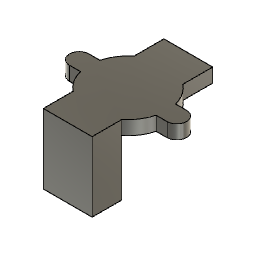
[new] Stepper Motor Cover v7 (Autodesk Fusion 360 design; units mm, degrees)
Autodesk Fusion 360 part; units mm, degrees
sketch "Sketch1" plane through (0, 0, 24.0553) normal (0, 0, 1) x (-1, 0, 0)
  line L0 (10.7499, 16.3506) -> (10.7499, 5.6583)
  line L1 (10.7499, 5.6583) -> (-6.7501, 5.6583)
  line L2 (-6.7501, 5.6583) -> (-6.7501, 16.3506)
  arc A0 (-11.5555, 23.7794) -> (-6.7501, 16.3506) centre (1.9999, 27.2794) ccw
  line L3 (-11.5555, 23.7794) -> (-15.5001, 23.7794)
  arc A1 (-15.5001, 30.7794) -> (-15.5001, 23.7794) centre (-15.5001, 27.2794) ccw
  line L4 (-15.5001, 30.7794) -> (-11.5555, 30.7794)
  arc A2 (-6.7501, 38.2081) -> (-11.5555, 30.7794) centre (1.9999, 27.2794) ccw
  line L5 (-6.7501, 38.2081) -> (-6.7501, 48.9005)
  line L6 (-6.7501, 48.9005) -> (10.7499, 48.9005)
  line L7 (10.7499, 48.9005) -> (10.7499, 38.2081)
  arc A3 (15.5554, 30.7794) -> (10.7499, 38.2081) centre (1.9999, 27.2794) ccw
  line L8 (15.5554, 30.7794) -> (19.4999, 30.7794)
  arc A4 (19.4999, 23.7794) -> (19.4999, 30.7794) centre (19.4999, 27.2794) ccw
  line L9 (19.4999, 23.7794) -> (15.5554, 23.7794)
  arc A5 (10.7499, 16.3506) -> (15.5554, 23.7794) centre (1.9999, 27.2794) ccw
  arc A6 (51.4999, 44.5294) -> (41.4999, 54.5294) centre (41.4999, 44.5294) ccw
  line L10 (41.4999, 54.5294) -> (-37.5001, 54.5294)
  arc A7 (-37.5001, 54.5294) -> (-47.5001, 44.5294) centre (-37.5001, 44.5294) ccw
  line L11 (-47.5001, 44.5294) -> (-47.5001, -34.4706)
  arc A8 (-47.5001, -34.4706) -> (-37.5001, -44.4706) centre (-37.5001, -34.4706) ccw
  line L12 (-37.5001, -44.4706) -> (41.4999, -44.4706)
  arc A9 (41.4999, -44.4706) -> (51.4999, -34.4706) centre (41.4999, -34.4706) ccw
  line L13 (51.4999, -34.4706) -> (51.4999, 44.5294)
  line L14 (42.9999, -37.9706) -> (-39.0001, -37.9706)
  line L15 (-39.0001, -37.9706) -> (-39.0001, 0.0294)
  line L16 (-39.0001, 0.0294) -> (42.9999, 0.0294)
  line L17 (42.9999, 0.0294) -> (42.9999, -37.9706)
  line L18 (10.7499, 48.9005) -> (10.7499, 38.2081)
  line L19 (-6.7501, 48.9005) -> (10.7499, 48.9005)
  line L20 (-6.7501, 38.2081) -> (-6.7501, 48.9005)
  arc A10 (-6.7501, 38.2081) -> (-11.5555, 30.7794) centre (1.9999, 27.2794) ccw
  arc A11 (15.5554, 30.7794) -> (10.7499, 38.2081) centre (1.9999, 27.2794) ccw
  line L21 (15.5554, 30.7794) -> (19.4999, 30.7794)
  arc A12 (19.4999, 23.7794) -> (19.4999, 30.7794) centre (19.4999, 27.2794) ccw
  line L22 (19.4999, 23.7794) -> (15.5554, 23.7794)
  arc A13 (15.5524, 23.7794) -> (15.5583, 30.7794) centre (1.9999, 27.2908) ccw
  line L23 (15.5524, 23.7794) -> (19.4999, 23.7794)
  arc A14 (19.4999, 23.7794) -> (19.4999, 30.7794) centre (19.4999, 27.2794) ccw
  line L24 (19.4999, 30.7794) -> (15.5583, 30.7794)
  circle A15 centre (19.4999, 27.2794) radius 2
  arc A16 (-11.5585, 30.7794) -> (-11.5526, 23.7794) centre (1.9999, 27.2908) ccw
  line L25 (-11.5585, 30.7794) -> (-15.5001, 30.7794)
  arc A17 (-15.5001, 30.7794) -> (-15.5001, 23.7794) centre (-15.5001, 27.2794) ccw
  line L26 (-15.5001, 23.7794) -> (-11.5526, 23.7794)
  circle A18 centre (-15.5001, 27.2794) radius 2
  line L27 (-6.7501, 5.6583) -> (-6.7501, 16.3506)
  line L28 (10.7499, 5.6583) -> (-6.7501, 5.6583)
  line L29 (10.7499, 16.3506) -> (10.7499, 5.6583)
  circle A19 centre (1.9999, 27.2908) radius 14
  arc A20 (-15.5001, 30.7794) -> (-15.5001, 23.7794) centre (-15.5001, 27.2794) ccw
  line L30 (-15.5001, 30.7794) -> (-11.5555, 30.7794)
  line L31 (-11.5555, 23.7794) -> (-15.5001, 23.7794)
  arc A21 (-11.5555, 23.7794) -> (-6.7501, 16.3506) centre (1.9999, 27.2794) ccw
  arc A22 (10.7499, 16.3506) -> (15.5554, 23.7794) centre (1.9999, 27.2794) ccw
  circle A23 centre (1.9999, 27.2908) radius 13
  circle A24 centre (19.4999, 27.2794) radius 1.5
  circle A25 centre (-15.5001, 27.2794) radius 1.5
extrude "Extrude2" add sketch "Sketch1" against normal blind 5 contours L0 L1 L2 A0 A5 L23 L26 L27 L28 L29 A19 A21 A22 | L8 A4 L9 L21 A12 L22 A13 L23 A14 L24 A19 | L4 A2 L5 L7 A3 L8 L18 L20 A10 A11 L21 A13 A16 A19 L30 | L3 A1 L4 A16 L25 A17 L26 A19 A20 L30 L31 | L7 A3 L8 L18 A11 L21 A19 | L4 A2 L5 L20 A10 A19 L30 | A23 makes body 1
extrude "Extrude1" add sketch "Sketch1" against normal blind 25 separate body contours L5 L6 L7 L18 L19 L20 A19 makes body 2
extrude "Extrude3" add sketch "Sketch1" against normal blind 4 separate body contours A15 | A18 makes body 3 at (-21.4974, -27.1797, 21.3887) makes body 4 at (13.5026, -27.1797, 21.3887)
sketch "Sketch2" plane through (0, 0, 24.0553) normal (0, 0, 1) x (-1, 0, 0)
  circle A0 centre (19.4999, 27.2794) radius 1.5
  circle A1 centre (19.4999, 27.2794) radius 1.5
  constraint concentric A0 A1
extrude "Extrude4" add sketch "Sketch2" against normal blind 2 bodies 3
sketch "Sketch3" plane through (0, 0, 24.0553) normal (0, 0, 1) x (-1, 0, 0)
  circle A0 centre (-15.5001, 27.2794) radius 1.5
  circle A1 centre (-15.5001, 27.2794) radius 1.5
  constraint concentric A0 A1
extrude "Extrude5" add sketch "Sketch3" against normal blind 2 bodies 4
extrude "Extrude6" add 1 faces at (13.7846, -26.6463, 20.0553) along direction (0, 0, -1) blind 1 on bodies 4 bodies 4 1
extrude "Extrude7" add 1 faces at (-18.7404, -28.9428, 20.0553) along direction (0, 0, -1) blind 1 on bodies 3 bodies 3 2 4
sketch "Sketch4" plane through (0, 0, 24.0553) normal (0, 0, 1) x (-1, 0, 0)
  line L0 (10.7499, 5.6583) -> (10.7499, 16.3506)
  arc A0 (10.7499, 16.3506) -> (15.5554, 23.7794) centre (1.9999, 27.2794) ccw
  line L1 (15.5554, 23.7794) -> (19.4999, 23.7794)
  arc A1 (19.4999, 23.7794) -> (19.4999, 30.7794) centre (19.4999, 27.2794) ccw
  line L2 (19.4999, 30.7794) -> (15.5554, 30.7794)
  arc A2 (15.5554, 30.7794) -> (10.7499, 38.2081) centre (1.9999, 27.2794) ccw
  line L3 (10.7499, 38.2081) -> (10.7499, 38.2196)
  arc A3 (10.7499, 38.2196) -> (-6.7501, 38.2196) centre (1.9999, 27.2908) ccw
  line L4 (-6.7501, 38.2196) -> (-6.7501, 38.2081)
  arc A4 (-6.7501, 38.2081) -> (-11.5555, 30.7794) centre (1.9999, 27.2794) ccw
  line L5 (-11.5555, 30.7794) -> (-15.5001, 30.7794)
  arc A5 (-15.5001, 30.7794) -> (-15.5001, 23.7794) centre (-15.5001, 27.2794) ccw
  line L6 (-15.5001, 23.7794) -> (-11.5555, 23.7794)
  arc A6 (-11.5555, 23.7794) -> (-6.7501, 16.3506) centre (1.9999, 27.2794) ccw
  line L7 (-6.7501, 16.3506) -> (-6.7501, 5.6583)
  line L8 (-6.7501, 5.6583) -> (10.7499, 5.6583)
  line L9 (10.7499, 48.9005) -> (-6.7501, 48.9005)
  line L10 (-6.7501, 48.9005) -> (-6.7501, 38.2196)
  arc A7 (10.7499, 38.2196) -> (-6.7501, 38.2196) centre (1.9999, 27.2908) ccw
  line L11 (10.7499, 38.2196) -> (10.7499, 48.9005)
  line L12 (10.7499, 38.2196) -> (10.7499, 48.9005)
  line L13 (-6.7501, 48.9005) -> (-6.7501, 38.2196)
  circle A8 centre (1.9999, 27.2908) radius 14
  constraint coincident L3.end A3.start
  constraint coincident L9.start L11.end
  constraint coincident L9.end L10.start
  constraint coincident A3.end L4.start
  constraint concentric A7 A8
  constraint coincident A3.end A8
extrude "Extrude8" add sketch "Sketch4" against normal blind 25 contours A3 L9 L10 A7 L11 L12 L13 A8 bodies 2 3
